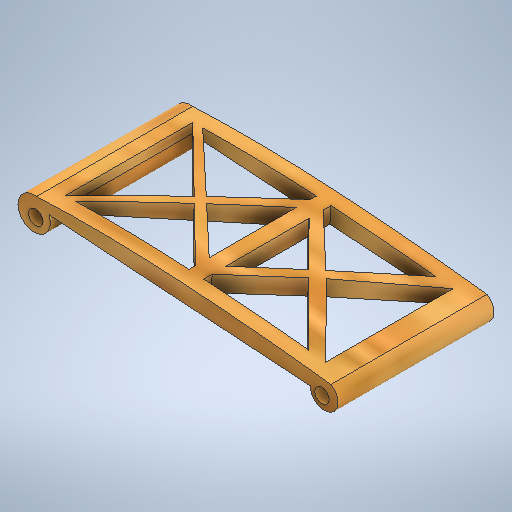
# Autodesk Inventor part: 2414 basic aerofoil
Saved by Autodesk Inventor 2025.1 (Build 291241000, 241)
## iProperties
Created: 2024-11-04
Part Number: 2414 basic aerofoil
Material: Plywood, Finish
Document SubType Name: Modeling
Designer: johan
Density: 0.552 g/cm^3
Appearance: Plywood - New
Author: johan
Autodesk Inventor part; units mm, degrees
ref_plane "YZ Plane" through (0, 0, 0) normal (1, 0, 0) x (0, 1, 0)
ref_plane "XZ Plane" through (0, 0, 0) normal (0, 1, 0) x (-1, 0, 0)
ref_plane "XY Plane" through (0, 0, 0) normal (0, 0, 1) x (1, 0, 0)
sketch "Sketch2" plane through (0, 0, 0) normal (0, 0, 1) x (1, 0, 0)
  spline S0 degree 5 number of poles 204
  circle A0 centre (79.5137, 4.5678) radius 15.1135
  line L0 (79.5137, 4.5678) -> (79.5137, -15.4763) construction
  line L1 (79.5137, 4.5678) -> (209.6498, 4.5678) construction
  line L2 (319.6498, 0.0573) -> (219.6498, 0.0573) construction
  line L3 (219.6499, 18.7671) -> (219.6499, 18.7671) construction
  line L4 (28.0055, 4.5054) -> (28.0055, -2.4946)
  line L5 (19.6272, 1.0326) -> (319.6498, 0.0573) construction
  line L6 (49.7105, 14.4213) -> (55.6079, 14.4213)
  line L7 (49.7104, -8.4915) -> (55.6078, -8.4915)
  line L8 (28.0055, 4.5054) -> (49.7105, 14.4213)
  line L9 (28.0055, -2.4946) -> (49.7104, -8.4915)
  line L10 (55.6079, 14.4213) -> (55.6079, 20.8729)
  line L11 (55.6078, -8.4915) -> (55.6078, -14.1513)
  line L12 (108.6496, 16.3299) -> (108.6496, -7.1942)
  line L13 (110.8735, -9.1817) -> (193.8736, 0.1678)
  line L14 (195.6498, 2.1552) -> (195.6498, 6.9805)
  arc A1 (108.6496, -7.1942) -> (110.8735, -9.1817) centre (110.6496, -7.1942) ccw
  arc A2 (193.8736, 0.1678) -> (195.6498, 2.1552) centre (193.6498, 2.1552) ccw
  circle A3 centre (209.6498, 0.0573) radius 6.214
  line L15 (108.6496, 18.5678) -> (195.6498, 8.7678)
  circle A4 centre (100.6496, 18.3866) radius 2.5
  circle A5 centre (199.6498, 14.5256) radius 2.5
  spline S1 degree 4 poles (202.7347, 19.3724) (199.838, 19.7251) (195.7649, 20.2061) (190.5032, 20.7952) (184.0435, 21.4697) (179.3239, 21.937) (174.5933, 22.3806) (169.8562, 22.7962) (165.1183, 23.1863) (160.3828, 23.5463) (155.6566, 23.8767) (150.936, 24.1762) (146.2498, 24.4444) (141.5311, 24.676) (136.9019, 24.8782) (132.2312, 25.0296) (127.6189, 25.1375) (123.0371, 25.1983) (118.5028, 25.2125) (112.3622, 25.1677) (107.3995, 25.0507) (103.5849, 24.9119) (100.8865, 24.7866) knots 0 0 0 0 0 0.114234 0.16008 0.206003 0.251978 0.297982 0.343994 0.389991 0.435949 0.481846 0.527693 0.573431 0.619092 0.664656 0.710064 0.755333 0.800383 0.845191 0.889734 1 1 1 1 1
  line L16 (105.191, 21.4637) -> (195.6498, 15.3862)
  arc A6 (100.8865, 24.7866) -> (105.191, 21.4637) centre (100.0416, 19.2427) ccw
  arc A7 (195.6498, 15.3862) -> (202.7347, 19.3724) centre (200.4212, 15.1951) ccw
  point P0 (0, 0)
  point P1 (319.5771, 0.0748)
  point P2 (319.3573, 0.1272)
  point P3 (318.9916, 0.2136)
  point P4 (318.4804, 0.3362)
  point P5 (317.8238, 0.4909)
  point P6 (317.0222, 0.6802)
  point P7 (316.0769, 0.9024)
  point P8 (314.9885, 1.1569)
  point P9 (313.7582, 1.443)
  point P10 (312.3866, 1.7598)
  point P11 (310.8752, 2.1063)
  point P12 (309.2258, 2.4819)
  point P13 (307.4393, 2.8854)
  point P14 (305.5178, 3.3153)
  point P15 (303.4628, 3.7707)
  point P16 (301.2764, 4.2501)
  point P17 (298.9607, 4.7526)
  point P18 (296.5175, 5.2764)
  point P19 (293.9492, 5.8203)
  point P20 (291.2585, 6.3828)
  point P21 (288.4478, 6.9627)
  point P22 (285.5195, 7.5582)
  point P23 (282.4766, 8.1678)
  point P24 (279.3218, 8.79)
  point P25 (276.0584, 9.4236)
  point P26 (272.6891, 10.0668)
  point P27 (269.2175, 10.7178)
  point P28 (265.6469, 11.3757)
  point P29 (261.9803, 12.0381)
  point P30 (258.2219, 12.7041)
  point P31 (254.3747, 13.3722)
  point P32 (250.4426, 14.0403)
  point P33 (246.4295, 14.7072)
  point P34 (242.339, 15.3714)
  point P35 (238.1756, 16.0311)
  point P36 (233.9428, 16.6851)
  point P37 (229.6454, 17.3316)
  point P38 (225.2869, 17.9694)
  point P39 (220.8723, 18.5967)
  point P40 (216.4049, 19.2123)
  point P41 (211.8901, 19.8144)
  point P42 (207.332, 20.4015)
  point P43 (202.7347, 20.9724)
  point P44 (198.1034, 21.5256)
  point P45 (193.4423, 22.0596)
  point P46 (188.7563, 22.5726)
  point P47 (184.0499, 23.0637)
  point P48 (179.3279, 23.5314)
  point P49 (174.5948, 23.9745)
  point P50 (169.8554, 24.3909)
  point P51 (165.1148, 24.7803)
  point P52 (160.3775, 25.1406)
  point P53 (155.6479, 25.4709)
  point P54 (150.9316, 25.7703)
  point P55 (146.233, 26.0373)
  point P56 (141.557, 26.2707)
  point P57 (136.8821, 26.4681)
  point P58 (132.2209, 26.6211)
  point P59 (127.5964, 26.7282)
  point P60 (123.0133, 26.7888)
  point P61 (118.4727, 26.8026)
  point P62 (113.9902, 26.7693)
  point P63 (109.5601, 26.6886)
  point P64 (105.191, 26.5611)
  point P65 (100.8865, 26.3866)
  point P66 (96.6524, 26.1647)
  point P67 (92.4927, 25.8975)
  point P68 (88.412, 25.5858)
  point P69 (84.409, 25.3061)
  point P70 (80.8803, 24.9766)
  point P71 (76.6761, 24.4558)
  point P72 (72.9631, 23.8932)
  point P73 (69.3402, 23.3612)
  point P74 (65.8208, 22.7938)
  point P75 (62.4086, 22.1884)
  point P76 (59.1071, 21.5462)
  point P77 (52.8493, 20.1606)
  point P78 (49.7107, 19.4213)
  point P79 (47.0737, 18.6508)
  point P80 (44.3741, 17.8542)
  point P81 (41.8033, 17.0323)
  point P82 (39.3638, 16.1875)
  point P83 (37.0582, 15.3214)
  point P84 (34.8883, 14.4364)
  point P85 (32.8567, 13.534)
  point P86 (30.9649, 12.6166)
  point P87 (29.2144, 11.686)
  point P88 (27.607, 10.7437)
  point P89 (26.1442, 9.7921)
  point P90 (24.8269, 8.8324)
  point P91 (23.6566, 7.8664)
  point P92 (22.6337, 6.8952)
  point P93 (21.7592, 5.9208)
  point P94 (21.0335, 4.944)
  point P95 (20.4573, 3.966)
  point P96 (20.031, 2.9874)
  point P97 (19.7541, 2.0097)
  point P98 (19.6496, 0.0598)
  point P99 (19.8207, -0.9032)
  point P100 (20.1378, -1.8356)
  point P101 (20.6004, -2.7401)
  point P102 (21.2081, -3.6158)
  point P103 (21.9599, -4.4627)
  point P104 (22.8545, -5.2806)
  point P105 (23.891, -6.069)
  point P106 (25.0682, -6.8277)
  point P107 (26.3845, -7.5561)
  point P108 (27.8383, -8.2539)
  point P109 (29.4283, -8.9211)
  point P110 (31.1522, -9.5571)
  point P111 (33.0086, -10.1613)
  point P112 (34.9949, -10.734)
  point P113 (37.1093, -11.2746)
  point P114 (39.3497, -11.7828)
  point P115 (41.7134, -12.2586)
  point P116 (44.1979, -12.702)
  point P117 (46.8014, -13.1127)
  point P118 (49.7105, -13.4915)
  point P119 (52.3532, -13.8357)
  point P120 (58.3469, -14.4294)
  point P121 (61.5023, -14.678)
  point P122 (64.7591, -14.8953)
  point P123 (68.1149, -15.0813)
  point P124 (71.5661, -15.237)
  point P125 (75.1094, -15.3627)
  point P126 (78.7418, -15.4596)
  point P127 (82.46, -15.528)
  point P128 (86.2607, -15.5691)
  point P129 (90.14, -15.5838)
  point P130 (94.0946, -15.5733)
  point P131 (98.1212, -15.5388)
  point P132 (102.2159, -15.4812)
  point P133 (106.3751, -15.4023)
  point P134 (110.5952, -15.303)
  point P135 (114.872, -15.1845)
  point P136 (119.2022, -15.0489)
  point P137 (123.5813, -14.8971)
  point P138 (128.006, -14.7306)
  point P139 (132.4718, -14.5509)
  point P140 (136.9748, -14.3598)
  point P141 (141.5285, -14.1576)
  point P142 (146.1365, -13.9383)
  point P143 (150.7679, -13.7022)
  point P144 (155.4191, -13.4499)
  point P145 (160.0853, -13.1829)
  point P146 (164.7617, -12.9024)
  point P147 (169.4444, -12.6099)
  point P148 (174.1283, -12.306)
  point P149 (178.8092, -11.9925)
  point P150 (183.4823, -11.67)
  point P151 (188.1434, -11.34)
  point P152 (192.7877, -11.0037)
  point P153 (197.4107, -10.6614)
  point P154 (202.0079, -10.3149)
  point P155 (206.5747, -9.9645)
  point P156 (211.1069, -9.6117)
  point P157 (215.5999, -9.2568)
  point P158 (220.0489, -8.9007)
  point P159 (224.4503, -8.5446)
  point P160 (228.7987, -8.1885)
  point P161 (233.0906, -7.8339)
  point P162 (237.3214, -7.4808)
  point P163 (241.4866, -7.1298)
  point P164 (245.5828, -6.7821)
  point P165 (249.6052, -6.4377)
  point P166 (253.5502, -6.0972)
  point P167 (257.4136, -5.7612)
  point P168 (261.1915, -5.4303)
  point P169 (264.88, -5.1051)
  point P170 (268.4758, -4.7856)
  point P171 (271.9747, -4.4724)
  point P172 (275.3734, -4.1661)
  point P173 (278.6686, -3.867)
  point P174 (281.8564, -3.5757)
  point P175 (284.9344, -3.2925)
  point P176 (287.8984, -3.018)
  point P177 (290.7463, -2.7525)
  point P178 (293.4745, -2.4963)
  point P179 (296.0806, -2.2503)
  point P180 (298.5616, -2.0142)
  point P181 (300.9151, -1.7892)
  point P182 (303.1387, -1.575)
  point P183 (305.23, -1.3728)
  point P184 (307.1866, -1.1823)
  point P185 (309.007, -1.0041)
  point P186 (310.6885, -0.8385)
  point P187 (312.2302, -0.6861)
  point P188 (313.6297, -0.5471)
  point P189 (314.8861, -0.4221)
  point P190 (315.9976, -0.3107)
  point P191 (316.9636, -0.214)
  point P192 (317.7826, -0.1311)
  point P193 (318.4538, -0.0643)
  point P194 (318.9765, -0.0102)
  point P195 (319.3503, 0.027)
  point P196 (319.5743, 0.0497)
  point P197 (28.0055, 1.0054)
  point P198 (108.6496, -9.4322)
  point P199 (195.6498, 0.3678)
  dimension "d37" = 30.227
  dimension "d2" = 300.0001
  dimension "d19" = 110
  dimension "d22" = 100
  dimension "d23" = 7
  dimension "d24" = 5
  dimension "d25" = 5
  dimension "d30" = 28
  dimension "d31" = 8.4
  dimension "d33" = 14
  dimension "d39" = 59.8865
  dimension "d42" = 12.428
  dimension "d43" = 5
  dimension "d44" = 5
  dimension "d49" = 1.6
  dimension "d50" = 1.6
  dimension "d51" = 1.6
  dimension "d52" = 1.6
  dimension "d53" = 1.6
  dimension "d54" = 1.6
  dimension "d55" = 1.6
  dimension "d56" = 1.6
  dimension "d57" = 1.6
  dimension "d58" = 1.6
  dimension "d59" = 1.6
  dimension "d60" = 1.6
  dimension "d61" = 1.6
  dimension "d62" = 1.6
  dimension "d63" = 1.6
  dimension "d64" = 1.6
  dimension "d65" = 1.6
  dimension "d66" = 1.6
  dimension "d67" = 1.6
  dimension "d68" = 1.6
  dimension "d69" = 1.6
  dimension "d70" = 1.6
  dimension "d72" = 1.6
  dimension "d75" = 4
  dimension "d76" = 7
  dimension "d90" = 8
  dimension "d91" = 8
  constraints: 34 end point, 10 point on line, 8 point on circle, 7 centre point, 5 vertical, 4 tangent, 3 midpoint, 2 horizontal, 2 horizontal alignment, 1 coincident, 1 parallel, 1 perpendicular, 278 other
  measures "d2" distance of L2.start point (19.65, 0.06)
  measures "d19" horizontal distance of L2.start L1.end
  measures "d22" distance of L2.start L2.end
  measures "d23" distance of L4.start L4.end
  measures "d24" distance from line of point (49.711, 19.421) L6
  measures "d25" distance from line of point (49.711, -13.491) L7
  measures "d30" distance of L15.start point (108.65, -9.432)
  measures "d31" distance of point (195.65, 0.368) L15.end
  measures "d33" distance from line of L1.end L14
  measures "d39" horizontal distance of L5.start L0.start
  measures "d42" diameter of A3
  measures "d43" diameter of A4
  measures "d44" diameter of A5
  measures "d49" distance of point (100.887, 26.387) A6.start
  measures "d50" distance of point (105.191, 26.561) point (105.191, 24.961)
  measures "d51" distance of point (109.56, 25.089) point (109.56, 26.689)
  measures "d52" distance of point (113.99, 25.169) point (113.99, 26.769)
  measures "d53" distance of point (118.476, 25.203) point (118.473, 26.803)
  measures "d54" distance of point (123.013, 25.189) point (123.013, 26.789)
  measures "d55" distance of point (127.596, 26.728) point (127.596, 25.128)
  measures "d56" distance of point (132.221, 25.021) point (132.221, 26.621)
  measures "d57" distance of point (136.882, 26.468) point (136.882, 24.868)
  measures "d58" vertical distance of point (141.557, 26.271) point (141.528, 24.671)
  measures "d59" distance of point (146.233, 24.437) point (146.233, 26.037)
  measures "d60" distance of point (150.932, 25.77) point (150.932, 24.17)
  measures "d61" distance of point (155.648, 25.471) point (155.648, 23.871)
  measures "d62" distance of point (160.377, 25.141) point (160.377, 23.541)
  measures "d63" distance of point (165.115, 24.78) point (165.115, 23.18)
  measures "d64" distance of point (169.855, 22.791) point (169.855, 24.391)
  measures "d65" distance of point (174.595, 22.375) point (174.595, 23.975)
  measures "d66" distance of point (179.328, 23.531) point (179.328, 21.931)
  measures "d67" distance of point (184.05, 23.064) point (184.05, 21.464)
  measures "d68" distance of point (188.756, 22.573) point (188.756, 20.973)
  measures "d69" distance of point (193.442, 20.46) point (193.442, 22.06)
  measures "d70" distance of point (198.103, 21.526) point (198.103, 19.926)
  measures "d72" distance of point (202.735, 20.972) A7.end
  measures "d75" distance from line of A5.centre L14
  measures "d76" vertical distance of point (198.103, 21.526) A5.centre
  measures "d90" vertical distance of point (100.887, 26.387) A4.centre
  measures "d91" horizontal distance of L15.start A4.centre
extrude "Extrusion8" add sketch "Sketch2" along normal blind 54 contours A7 L16 A6 S1
sketch "Sketch3" plane through (195.6498, 15.3862, 0) normal (-0.067, -0.9978, 0) x (0.9978, -0.067, 0)
  line L0 (-0.0017, 49) -> (-0.0017, 5)
  line L1 (-0.0017, 5) -> (-22.7277, 26.2297)
  line L2 (-22.7277, 26.2297) -> (-0.0017, 49)
  line L3 (-67.7277, 27.0011) -> (-45.2277, 49.0011)
  line L4 (-45.2277, 49.0011) -> (-45.2277, 5.0011)
  line L5 (-45.2277, 5.0011) -> (-67.7277, 27.0011)
  line L6 (-45.2277, 49.0011) -> (-22.7277, 26.2297)
  line L7 (-45.2277, 5.0011) -> (-22.7277, 26.2297)
  line L8 (9.5487, 54) -> (0, 54) projected
  line L9 (9.5487, 0) -> (0, 0) projected
  line L10 (-90.2837, 49) -> (-90.1718, 5)
  line L11 (-90.1718, 5) -> (-67.7277, 27.0011)
  line L12 (-90.2837, 49) -> (-67.7277, 27.0011)
  line L13 (-90.0437, 54) -> (-101.2596, 54) projected
  line L14 (-90.0437, 0) -> (-101.2596, 0) projected
  line L15 (-90.2837, 49) -> (-0.0017, 49)
  line L16 (-0.0017, 5) -> (-90.1718, 5)
  line L17 (-86.7403, 49) -> (-45.0868, 9.6057)
  line L18 (-86.7403, 5) -> (-45.2277, 44.1668)
  line L19 (-45.2277, 44.1668) -> (-5.985, 5)
  line L20 (-5.985, 49) -> (-45.2277, 9.739)
  line L21 (-47.5072, 5) -> (-47.5072, 49)
  line L22 (-42.3779, 49) -> (-42.3779, 5)
  point P0 (-194.1783, 0)
  point P1 (-90.6627, 0)
  point P2 (-45.2277, 27.0011)
  point P3 (6.8018, 54)
  point P4 (6.8018, 0)
  point P5 (-95.1802, 54)
  point P6 (-90.6627, 54)
  point P7 (-95.1802, 0)
  point P8 (-28.0012, 26.9736)
  point P9 (-63.4507, 26.9736)
  point P10 (-25.7189, 29.2569)
  point P11 (-45.2266, 49)
  point P12 (-65.6391, 29.0433)
  point P13 (-45.2288, 49)
  point P14 (-25.0554, 24.0335)
  point P15 (-65.6131, 24.9334)
  point P16 (-42.3779, 7.6899)
  point P17 (-42.3779, 41.3225)
  point P18 (-42.3779, 12.5902)
  point P19 (-42.3779, 46.1169)
  point P20 (-47.5072, 46.7723)
  point P21 (-47.5072, 7.23)
  point P22 (-47.5072, 11.8949)
  point P23 (-47.5072, 42.0161)
  dimension "d81" = 22.5
  dimension "d82" = 22.5
  dimension "d83" = 5
  dimension "d84" = 5
  dimension "d85" = 22.5
  dimension "d86" = 5
  dimension "d87" = 5
  constraints: 38 end point, 11 point on line, 2 parallel, 2 vertical, 1 midpoint, 1 perpendicular
  measures "d81" distance of point (-45.228, 27.001) L3.start
  measures "d82" distance from line of L1.end L4
  measures "d83" distance from line of L8 L0.start
  measures "d84" distance from line of L9 L0.end
  measures "d85" distance from line of L10 L3.start
  measures "d86" distance from line of L13 L10.start
  measures "d87" distance from line of L14 L10.end
extrude "Extrusion9" cut sketch "Sketch3" against normal blind 10 contours L0 L1 L2 | L20 L6 L22 L15 | L16 L22 L7 L19 | L20 L22 L19 | L3 L17 L15 L21 | L21 L16 L18 L5 | L21 L17 L18 | L11 L10 L12
body "Solid8"
